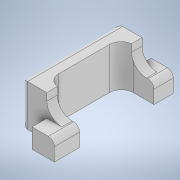
# Autodesk Inventor part: Button
Saved by Autodesk Inventor 2020.1 (Build 241239000, 239)
## iProperties
Created: 2021-08-24
Part Number: Button
Material: Generic
Document SubType Name: Modeling
Designer: nigel
Density: 1 g/cm^3
Appearance: Default
Author: nigel
Autodesk Inventor part; units mm, degrees
ref_plane "YZ Plane" through (0, 0, 0) normal (1, 0, 0) x (0, 1, 0)
ref_plane "XZ Plane" through (0, 0, 0) normal (0, 1, 0) x (-1, 0, 0)
ref_plane "XY Plane" through (0, 0, 0) normal (0, 0, 1) x (1, 0, 0)
sketch "Sketch1" plane through (0, 0, 0) normal (0, 1, 0) x (-1, 0, 0)
  line L0 (0.85, 3.2) -> (-0.85, 3.2)
  line L1 (-0.85, 3.2) -> (-0.85, -3.2)
  line L2 (-0.85, -3.2) -> (0.85, -3.2)
  line L3 (0.85, -3.2) -> (0.85, 3.2)
  line L4 (0.85, 3.2) -> (-0.85, -3.2) construction
  line L5 (-0.85, 3.2) -> (0.85, -3.2) construction
  line L6 (-0.85, -1.3) -> (-2.35, -1.3) construction
  line L7 (-2.35, -1.3) -> (-2.35, -3.4525)
  line L8 (-0.85, -3.2) -> (-0.85, -1.3)
  line L9 (-2.35, -3.4525) -> (-2.35, -3.8)
  line L10 (-2.35, -3.8) -> (-0.85, -3.8)
  line L11 (-0.85, -3.8) -> (-0.85, -3.2)
  line L12 (-2.35, -2.5) -> (-0.85, -2.5)
  line L13 (0, 0) -> (-4.1965, 0) construction
  line L14 (-2.35, 1.3) -> (-2.35, 3.4525)
  line L15 (-2.35, 2.5) -> (-0.85, 2.5)
  line L16 (-0.85, 2.5) -> (-2.35, 2.5)
  line L17 (-2.35, 2.5) -> (-2.35, 4.2)
  line L18 (-2.35, 4.2) -> (-0.85, 4.2)
  line L19 (-0.85, 4.2) -> (-0.85, 2.5)
  line L20 (-0.85, 2.5) -> (-0.15, 2.5)
  line L21 (-0.15, 2.5) -> (-0.15, -2.5)
  line L22 (-0.15, -2.5) -> (-0.85, -2.5)
  line L23 (-0.85, -2.5) -> (-0.85, 2.5)
  point P0 (-0.85, 2.5)
  point P1 (-0.85, -2.5)
  point P2 (-2.35, 3.4525)
  dimension "d0" = 1.3
  dimension "d2" = 1.7
  dimension "d3" = 1.5
  dimension "d5" = 1.9
  dimension "d7" = 2.5
  dimension "d13" = 1
  dimension "d14" = 2.5
  dimension "d18" = 0.7
  constraints: 48 end point, 8 parallel, 6 point on line, 5 horizontal, 5 perpendicular, 4 symmetric about line, 2 midpoint, 1 collinear, 1 vertical
  measures "d0" distance from line of L13.start L6
  measures "d2" distance between parallel lines of L3 L1
  measures "d3" distance between parallel lines of L1 L7
  measures "d5" distance between parallel lines of L2 L6
  measures "d7" distance from line of L13.start L12
  measures "d13" distance between parallel lines of L0 L18
  measures "d14" distance between parallel lines of L6 L10
  measures "d18" distance of L15.end L20.end
extrude "Extrusion1" add sketch "Sketch1" along normal blind 2.8 contours L3 L2 L1 L22 L21 L20 L0 | L1 L15 L14 L17 L18 L19 | L11 L10 L9 L7 L12 L1
sketch "Sketch2" plane through (0, 0, 0) normal (0, 0, 1) x (1, 0, 0)
  line L0 (0.85, 2.8) -> (2.35, 2.8)
  line L1 (2.35, 2.8) -> (2.35, 1.3)
  line L2 (2.35, 1.3) -> (0.85, 1.3)
  line L3 (0.85, 1.3) -> (0.85, 2.8)
  line L4 (2.35, 0) -> (2.35, 2.8) projected
  line L5 (0.85, 0) -> (0.85, 2.8) projected
  line L6 (0.85, 2.8) -> (2.35, 2.8) projected
  dimension "d15" = 1.5
  constraints: 8 end point, 2 coincident, 2 collinear, 2 parallel, 1 horizontal, 1 perpendicular, 1 point on line
  measures "d15" distance of L0.end L1.end
extrude "Extrusion2" cut sketch "Sketch2" along normal through all both and the other way through all
fillet "Fillet1" radius 0.8 2 edges at (0.15, 1.4, -2.5) (0.15, 1.4, 2.5)
fillet "Fillet1" radius 1 2 edges at (0.85, 1.3, 2.85) (0.85, 1.3, -2.85)
fillet "Fillet1" radius 0.4 2 edges at (2.35, 1.3, 3.35) (2.35, 1.3, -3.15)
fillet "Fillet1" radius 0.4 4 edges at (-0.85, 2.8, 0) (-0.85, 0, 0) (-0.85, 1.4, -3.2) (-0.85, 1.4, 3.2)
equation "\"button_height\" = 1.3"
body "Solid1"
